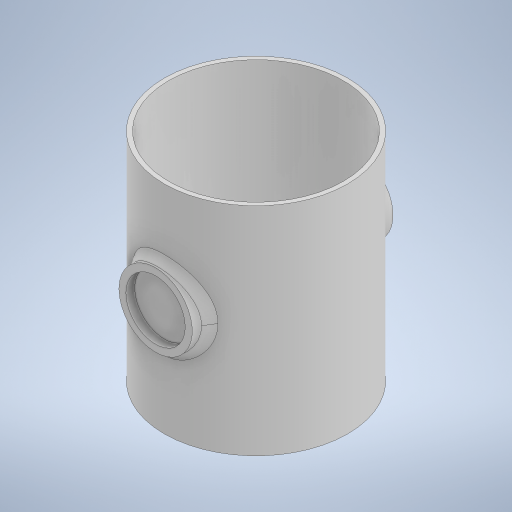
# Autodesk Inventor part: container
Saved by Autodesk Inventor 2024.2 (Build 282272000, 272)
## iProperties
Created: 2024-03-15
Part Number: container
Material: Generic
Document SubType Name: Sheet Metal
Designer: ellix
Density: 1 g/cm^3
Sheet Metal Rule: Default_mm
Appearance: Default
Author: ellix
Autodesk Inventor part; units mm, degrees
ref_plane "YZ Plane" through (0, 0, 0) normal (1, 0, 0) x (0, 1, 0)
ref_plane "XZ Plane" through (0, 0, 0) normal (0, 1, 0) x (-1, 0, 0)
sketch "Sketch1" plane through (0, 0, 0) normal (0, 1, 0) x (-1, 0, 0)
  circle A0 centre (0, 0) radius 25
  circle A1 centre (0, 0) radius 26.25
  dimension "d0" = 50
  dimension "d1" = 52.5
  constraints: 2 centre point, 2 coincident
  measures "d0" diameter of A0
  measures "d1" diameter of A1
extrude "Extrusion1" add sketch "Sketch1" along normal blind 60
sketch "Sketch2" plane through (0, 0, 0) normal (0, 0, 1) x (1, 0, 0)
  line L0 (26.25, 60) -> (-26.25, 60) projected
  line L1 (26.25, 0) -> (-26.25, 0) projected
  circle A0 centre (0, 30) radius 8.5
  circle A1 centre (0, 30) radius 10.5
  circle A2 centre (0, 30) radius 11.75
  point P0 (0, 0)
  point P1 (-1.1573, 60)
  point P2 (1.1573, 60)
  dimension "d4" = 17
  dimension "d5" = 21
  dimension "d10" = 23.5
  dimension "d15" = 30
  dimension "d16" = 60
  constraints: 3 centre point, 2 coincident
  measures "d4" diameter of A0
  measures "d5" diameter of A1
  measures "d10" diameter of A2
  measures "d15" distance from line of A2.centre L0
  measures "d16" distance between parallel lines of L1 L0
extrude "Extrusion2" add sketch "Sketch2" along normal mid plane 60 contours A1
sketch "Sketch3" plane through (0, 0, 0) normal (0, 1, 0) x (-1, 0, 0)
  point P0 (0, 0)
sketch "Sketch6" plane through (0, 0, 0) normal (0, 1, 0) x (-1, 0, 0)
  circle A0 centre (0, 0) radius 25 projected
extrude "Extrusion7" cut sketch "Sketch6" along normal blind 52.5
sketch "Sketch7" plane through (0, 0, 0) normal (0, -1, 0) x (1, 0, 0)
  circle A0 centre (0, 0) radius 26.25 projected
extrude "Extrusion8" add sketch "Sketch7" along normal blind 2
sketch "Sketch8" plane through (0, -2, 0) normal (0, -1, 0) x (1, 0, 0)
  circle A0 centre (0, 0) radius 28.75
  line L0 (-26.314, 28.75) -> (25.0961, 28.75)
  line L1 (25.0961, 28.75) -> (25.0961, -28.75)
  line L2 (25.0961, -28.75) -> (-26.314, -28.75)
  line L3 (-26.314, -28.75) -> (-26.314, 28.75)
  line L4 (-43.3732, 38.0408) -> (45.5671, 38.0408)
  line L5 (45.5671, 38.0408) -> (45.5671, -49.4262)
  line L6 (45.5671, -49.4262) -> (-43.3732, -49.4262)
  line L7 (-43.3732, -49.4262) -> (-43.3732, 38.0408)
  point P0 (-26.314, 11.5816)
  point P1 (25.0961, 14.0267)
  point P2 (25.0961, -14.0267)
  point P3 (-26.314, -11.5816)
  dimension "d23" = 57.5
  constraints: 16 end point, 4 parallel, 2 horizontal, 2 perpendicular, 1 centre point, 1 coincident
  measures "d23" diameter of A0
extrude "Extrusion9" cut sketch "Sketch8" against normal blind 64.5
sketch "Sketch9" plane through (0, 0, 0) normal (0, 1, 0) x (-1, 0, 0)
  circle A0 centre (0, 0) radius 26.25 projected
  line L0 (0, -26.25) -> (0, -28.75)
  line L1 (10.5, -28.75) -> (-10.5, -28.75) projected
  constraints: 2 end point, 1 midpoint, 1 vertical alignment, 1 other
ref_plane "Work Plane2" through (0, 0, -26.25) normal (0, 0, -1) x (-1, 0, 0)
sketch "Sketch10" plane through (0, 0, -26.25) normal (0, 0, -1) x (-1, 0, 0)
  spline S0 degree 5 poles (-8.5, 30) (-8.5, 31.1048) (-8.3205, 32.207) (-7.9633, 33.286) (-7.4183, 34.3212) (-6.1165, 35.9698) (-5.4477, 36.6272) (-4.6552, 37.2193) (-3.7372, 37.7125) (-1.6975, 38.3954) (-0.581, 38.5963) (0.581, 38.5963) (1.6975, 38.3954) (3.7372, 37.7125) (4.6552, 37.2193) (5.4477, 36.6272) (6.1165, 35.9698) (7.4183, 34.3212) (7.9633, 33.286) (8.3205, 32.207) (8.5, 31.1048) (8.5, 29.1432) (8.3921, 28.2874) (8.1764, 27.4417) (7.8503, 26.6182) (6.9783, 25.0684) (6.4394, 24.3403) (5.7823, 23.6583) (4.9996, 23.0472) (3.3803, 22.1598) (2.5864, 21.8333) (1.7239, 21.6031) (0.8192, 21.4903) (-0.9701, 21.5103) (-1.8319, 21.6326) (-2.6524, 21.8607) (-3.4091, 22.1756) (-4.7277, 22.8981) (-5.3057, 23.3049) (-5.8205, 23.7523) (-6.2744, 24.2302) (-7.4183, 25.6788) (-7.9633, 26.714) (-8.3205, 27.793) (-8.5, 28.8952) (-8.5, 30) knots 0 0 0 0 0 0 0.11918 0.11918 0.11918 0.11918 0.207551 0.207551 0.207551 0.207551 0.292734 0.292734 0.292734 0.292734 0.381106 0.381106 0.381106 0.381106 0.500285 0.500285 0.500285 0.500285 0.592715 0.592715 0.592715 0.592715 0.682548 0.682548 0.682548 0.682548 0.751759 0.751759 0.751759 0.751759 0.818053 0.818053 0.818053 0.818053 0.881099 0.881099 0.881099 0.881099 1 1 1 1 1 1 projected
  point P0 (0, 0)
  constraints: 1 other
extrude "Extrusion10" add sketch "Sketch10" against normal blind 52.5
sketch "Sketch11" plane through (0, 0, 0) normal (0, 1, 0) x (1, 0, 0)
  circle A0 centre (0, 0) radius 25 projected
extrude "Extrusion11" cut sketch "Sketch11" along normal blind 85.25
chamfer "Chamfer1" distance 2 angle 45 2 edges at (-10.5, 30.0261, -24.0585) (-10.5, 30.0261, 24.0585)
equation "\"BendRadius\" = Thickness"
equation "\"BendReliefWidth\" = Thickness"
equation "\"BendReliefDepth\" = 0.5 * Thickness"
equation "\"CornerReliefSize\" = 4 * Thickness"
equation "\"MinimumRemnant\" = 2 * Thickness"
equation "\"TransitionRadius\" = BendRadius"
equation "\"JacobiRadiusSize\" = BendRadius"
equation "\"GapSize\" = Thickness"
equation "\"Thickness\" = 0.5"
body "Solid1"
